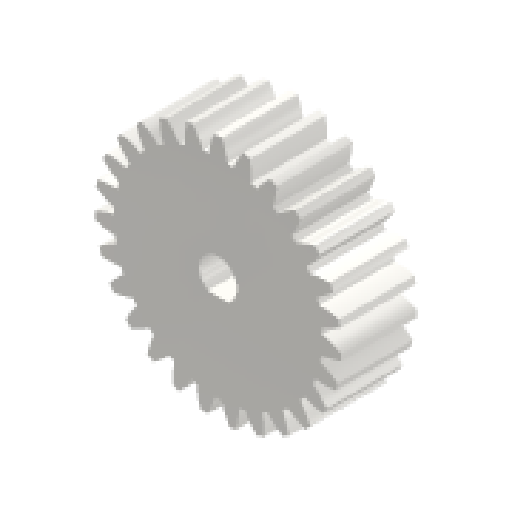
# Autodesk Inventor part: Stirnzahnrad1
Saved by Autodesk Inventor 2024.1 (Build 281209000, 209)
## iProperties
Created: 2024-04-15
Part Number: Stirnzahnrad1
Material: Steel
Document SubType Name: Modeling
Designer: diederichbenedict
Categories: <?xml version="1.0" encoding="UTF-16"?> <MemberInstance><Categories><FamilyTemplate><FamilyTemplateParameter ValueType="xs:double" Id="1" ObjectReferenceKey="da_z" ObjectType="kUserParameterObject"/><FamilyTemplateParameter ValueType="xs:double" Id="2" ObjectReferenceKey="da_b" ObjectType="kUserParameterObject"/><FamilyTemplateParameter ValueType="xs:double" Id="3" ObjectReferenceKey="da_beta" ObjectType="kUserParameterObject"/><FamilyTemplateParameter ValueType="xs:double" Id="4" ObjectReferenceKey="da_da" ObjectType="kUserParameterObject"/><FamilyTemplateParameter ValueType="xs:double" Id="5" ObjectReferenceKey="da_aw" ObjectType="kUserParameterObject"/><FamilyTemplateParameter ValueType="xs:string" Id="6" ObjectReferenceKey="EAIAABAAAACIAQAAAAAAAIAAAAAAAAAA" ObjectType="83910656" SubObjectId="SurfaceGeometry"/></FamilyTemplate><ParamToTemplateMap><ParamToTemplate CategoryParameter="//CategoryParameter[@InternalName='046C89C9-8512-4d59-83FE-43B91F4F132A']" TemplateParameter="1"/><ParamToTemplate CategoryParameter="//CategoryParameter[@InternalName='2552DF32-E462-4b46-AEBF-C6C7768E72AC']" TemplateParameter="2"/><ParamToTemplate CategoryParameter="//CategoryParameter[@InternalName='C9EE641D-15FC-4fae-A226-E94C4372FDD7']" TemplateParameter="3"/><ParamToTemplate><ParamToTemplate CategoryParameter="//CategoryParameter[@InternalName='00B6519A-459B-49c7-AD84-2E56D39A5744']" ConstantValue="0.000000"/></ParamToTemplate><ParamToTemplate><ParamToTemplate CategoryParameter="//CategoryParameter[@InternalName='04B31F0E-C7A6-4894-AA32-9629BEFACF47']" ConstantValue="1.000000"/></ParamToTemplate><ParamToTemplate><ParamToTemplate CategoryParameter="//CategoryParameter[@InternalName='43CBEC2E-7847-49e7-A936-2F7889FCB2D9']" ConstantValue="0.250000"/></ParamToTemplate><ParamToTemplate><ParamToTemplate CategoryParameter="//CategoryParameter[@InternalName='B1EFC894-105D-4ebd-86BF-FA20ED196853']" ConstantValue="0.350000"/></ParamToTemplate><ParamToTemplate><ParamToTemplate CategoryParameter="//CategoryParameter[@InternalName='51175063-3D10-4879-93E8-6246FE8B403D']" ConstantValue="2060000000.000000"/></ParamToTemplate><ParamToTemplate><ParamToTemplate CategoryParameter="//CategoryParameter[@InternalName='A3A52E27-4454-46a9-B0BD-C932399B70AF']" ConstantValue="0.300000"/></ParamToTemplate><ParamToTemplate><ParamToTemplate CategoryParameter="//CategoryParameter[@InternalName='91B76062-C214-41d9-B1B9-14D2AB99603D']" ConstantValue="0.112500"/></ParamToTemplate><ParamToTemplate><ParamToTemplate CategoryParameter="//CategoryParameter[@InternalName='374E806E-8B8A-4dda-A9AA-1039D6500AD2']" ConstantValue="8.888889"/></ParamToTemplate><ParamToTemplate><ParamToTemplate CategoryParameter="//CategoryParameter[@InternalName='2D373A89-B862-43d6-8D0B-0CBF12AB9F6C']" ConstantValue="0.349066"/></ParamToTemplate><ParamToTemplate CategoryParameter="//CategoryParameter[@InternalName='37777632-D6A2-4fac-9D53-DB8ACD95C989']" TemplateParameter="4"/><ParamToTemplate CategoryParameter="//CategoryParameter[@InternalName='FD1017F1-B727-4f7e-9707-0F86F1FF9423']" TemplateParameter="5"/><ParamToTemplate><ParamToTemplate CategoryParameter="//CategoryParameter[@InternalName='9E1B4470-B2D3-4ff1-B813-535BB4CDF51A']" ConstantValue="3520000.000000"/></ParamToTemplate><ParamToTemplate><ParamToTemplate CategoryParameter="//CategoryParameter[@InternalName='F8452263-BFF6-458c-9FB1-07C4B99E95CD']" ConstantValue="11400000.000000"/></ParamToTemplate><ParamToTemplate><ParamToTemplate CategoryParameter="//CategoryParameter[@InternalName='3E3BB259-FD49-497f-8171-6EBC954A3479']" ConstantValue="2.000000"/></ParamToTemplate><ParamToTemplate CategoryParameter="//CategoryParameter[@InternalName='27C3BAF2-7550-4e4b-AE2C-0DB134B7D9B7']" TemplateParameter="6"/></ParamToTemplateMap><Category DisplayName="Gear" InternalName="DC85795E-93AB-48d5-8EEE-5A27447B64BD" Mnemonic="Gear"><CategoryParameter DisplayName="z" InternalName="046C89C9-8512-4d59-83FE-43B91F4F132A" Mnemonic="z"/><CategoryParameter DisplayName="b" InternalName="2552DF32-E462-4b46-AEBF-C6C7768E72AC" Mnemonic="b"/><CategoryParameter DisplayName="||b|" InternalName="C9EE641D-15FC-4fae-A226-E94C4372FDD7" Mnemonic="beta"/><CategoryParameter DisplayName="x" InternalName="00B6519A-459B-49c7-AD84-2E56D39A5744" Mnemonic="x"/><CategoryParameter DisplayName="a*" InternalName="04B31F0E-C7A6-4894-AA32-9629BEFACF47" Mnemonic="a"/><CategoryParameter DisplayName="c*" InternalName="43CBEC2E-7847-49e7-A936-2F7889FCB2D9" Mnemonic="c"/><CategoryParameter DisplayName="r|.f|*" InternalName="B1EFC894-105D-4ebd-86BF-FA20ED196853" Mnemonic="rf"/><CategoryParameter DisplayName="E" InternalName="51175063-3D10-4879-93E8-6246FE8B403D" Mnemonic="E"/><CategoryParameter DisplayName="||m|" InternalName="A3A52E27-4454-46a9-B0BD-C932399B70AF" Mnemonic="mi"/><Category DisplayName="SpurGear" InternalName="26C5A22E-A91E-4dfd-A3B3-23CCAFAE1764" Mnemonic="SpurGear"><CategoryParameter DisplayName="m" InternalName="91B76062-C214-41d9-B1B9-14D2AB99603D" Mnemonic="m"/><CategoryParameter DisplayName="P" InternalName="374E806E-8B8A-4dda-A9AA-1039D6500AD2" Mnemonic="PP"/><CategoryParameter DisplayName="||a|" InternalName="2D373A89-B862-43d6-8D0B-0CBF12AB9F6C" Mnemonic="alpha"/><CategoryParameter DisplayName="d|.a|" InternalName="37777632-D6A2-4fac-9D53-DB8ACD95C989" Mnemonic="da"/><CategoryParameter DisplayName="a|.w|" InternalName="FD1017F1-B727-4f7e-9707-0F86F1FF9423" Mnemonic="aw"/><CategoryParameter DisplayName="||s||.Flim|" InternalName="9E1B4470-B2D3-4ff1-B813-535BB4CDF51A" Mnemonic="sFlim"/><CategoryParameter DisplayName="||s||.Hlim|" InternalName="F8452263-BFF6-458c-9FB1-07C4B99E95CD" Mnemonic="sHlim"/><CategoryParameter DisplayName="Typ" InternalName="3E3BB259-FD49-497f-8171-6EBC954A3479" Mnemonic="type"/><CategoryParameter DisplayName="PitchDiameter" InternalName="27C3BAF2-7550-4e4b-AE2C-0DB134B7D9B7" Mnemonic="IDS_PITCHDIAM"/></Category></Category></Categories></MemberInstance>
Density: 1 g/cm^3
Appearance: Steel
CustomPartVersion: 1
Author: diederichbenedict
Autodesk Inventor part; units mm, degrees
sketch "Sketch1" plane through (0, 0, 0) normal (0, 0, 1) x (1, 0, 0)
  circle A0 centre (0, 0) radius 16.3108
  dimension "d0" = 32.6217
  constraints: 1 centre point
  measures "d0" diameter of A0
extrude "Extrusion1" add sketch "Sketch1" along normal blind 10
ref_plane "Work Plane2" through (0, 0, 5) normal (0, 0, 1) x (1, 0, 0)
sketch "Sketch2" plane through (0, 0, 0) normal (0, 0, -1) x (-1, 0, 0)
  circle A0 centre (0, 0) radius 16.3108 projected
  circle A1 centre (0, 0) radius 15.1875
  dimension "d3" = 30.375
  constraints: 1 centre point, 1 coincident
  measures "d3" diameter of A1
surface extrude "Flankendurchmesser" sketch "Sketch2" against normal through all shown no curves A1
ref_plane "Work Plane8" through (0, 0, 0) normal (0.9932384, 0.1160929, 0) x (0, 0, 1)
ref_plane "Work Plane9" through (0, 0, 0) normal (1, 0, 0) x (0, 1, 0)
spur gear teeth "Stirnzahnrad" teeth 27 pitch diameter 30.375 tip diameter 32.6217 root diameter 27.5625 face width 20 start plane through (0, 0, 0) normal (0, 0, -1) x (-1, 0, 0)
sketch "Skizze3" plane through (0, 0, 10) normal (0, 0, 1) x (1, 0, 0)
  arc A0 (-4.2216, 15.7551) -> (-4.3348, 13.0818) centre (6.3804, 13.9668) ccw projected
  arc A1 (-4.3348, 13.0818) -> (-5.0881, 12.8076) centre (0, 0) ccw projected
  arc A2 (-5.0881, 12.8076) -> (-6.8933, 14.7826) centre (-13.8653, 6.598) ccw projected
  arc A3 (-6.8933, 14.7826) -> (-7.7411, 14.3568) centre (0, 0) ccw projected
  arc A4 (-7.7411, 14.3568) -> (-7.2348, 11.7295) centre (2.9874, 15.0617) ccw projected
  arc A5 (-7.2348, 11.7295) -> (-7.9046, 11.2889) centre (0, 0) ccw projected
  arc A6 (-7.9046, 11.2889) -> (-10.1166, 12.7945) centre (-15.0132, 3.2225) ccw projected
  arc A7 (-10.1166, 12.7945) -> (-10.8434, 12.1846) centre (0, 0) ccw projected
  arc A8 (-10.8434, 12.1846) -> (-9.7448, 9.7448) centre (-0.5666, 15.3447) ccw projected
  arc A9 (-9.7448, 9.7448) -> (-10.2949, 9.1617) centre (0, 0) ccw projected
  arc A10 (-10.2949, 9.1617) -> (-12.7945, 10.1166) centre (-15.3517, -0.3266) ccw projected
  arc A11 (-12.7945, 10.1166) -> (-13.361, 9.3555) centre (0, 0) ccw projected
  arc A12 (-13.361, 9.3555) -> (-11.7295, 7.2348) centre (-4.09, 14.8004) ccw projected
  arc A13 (-11.7295, 7.2348) -> (-12.1303, 6.5406) centre (0, 0) ccw projected
  arc A14 (-12.1303, 6.5406) -> (-14.7826, 6.8933) centre (-14.8626, -3.8581) ccw projected
  arc A15 (-14.7826, 6.8933) -> (-15.1584, 6.0221) centre (0, 0) ccw projected
  arc A16 (-15.1584, 6.0221) -> (-13.0818, 4.3348) centre (-7.393, 13.4583) ccw projected
  arc A17 (-13.0818, 4.3348) -> (-13.3117, 3.5668) centre (0, 0) ccw projected
  arc A18 (-13.3117, 3.5668) -> (-15.9739, 3.2983) centre (-13.5722, -7.1817) ccw projected
  arc A19 (-15.9739, 3.2983) -> (-16.1386, 2.364) centre (0, 0) ccw projected
  arc A20 (-16.1386, 2.364) -> (-13.7288, 1.2011) centre (-10.2974, 11.3905) ccw projected
  arc A21 (-13.7288, 1.2011) -> (-13.7754, 0.4008) centre (0, 0) ccw projected
  arc A22 (-13.7754, 0.4008) -> (-16.3039, -0.4744) centre (-11.5501, -10.1181) ccw projected
  arc A23 (-16.3039, -0.4744) -> (-16.2488, -1.4216) centre (0, 0) ccw projected
  arc A24 (-16.2488, -1.4216) -> (-13.6357, -1.9973) centre (-12.6467, 8.7088) ccw projected
  arc A25 (-13.6357, -1.9973) -> (-13.4965, -2.7868) centre (0, 0) ccw projected
  arc A26 (-13.4965, -2.7868) -> (-15.7551, -4.2216) centre (-8.9054, -12.509) ccw projected
  arc A27 (-15.7551, -4.2216) -> (-15.4829, -5.1305) centre (0, 0) ccw projected
  arc A28 (-15.4829, -5.1305) -> (-12.8076, -5.0881) centre (-14.3142, 5.5575) ccw projected
  arc A29 (-12.8076, -5.0881) -> (-12.4901, -5.8242) centre (0, 0) ccw projected
  arc A30 (-12.4901, -5.8242) -> (-14.3568, -7.7411) centre (-5.7806, -14.2255) ccw projected
  arc A31 (-14.3568, -7.7411) -> (-13.8824, -8.5628) centre (0, 0) ccw projected
  arc A32 (-13.8824, -8.5628) -> (-11.2889, -7.9046) centre (-15.21, 2.1066) ccw projected
  arc A33 (-11.2889, -7.9046) -> (-10.8102, -8.5476) centre (0, 0) ccw projected
  arc A34 (-10.8102, -8.5476) -> (-12.1846, -10.8434) centre (-2.3441, -15.1752) ccw projected
  arc A35 (-12.1846, -10.8434) -> (-11.5335, -11.5335) centre (0, 0) ccw projected
  arc A36 (-11.5335, -11.5335) -> (-9.1617, -10.2949) centre (-15.2858, -1.4578) ccw projected
  arc A37 (-9.1617, -10.2949) -> (-8.5476, -10.8102) centre (0, 0) ccw projected
  arc A38 (-8.5476, -10.8102) -> (-9.3555, -13.361) centre (1.2187, -15.3067) ccw projected
  arc A39 (-9.3555, -13.361) -> (-8.5628, -13.8824) centre (0, 0) ccw projected
  arc A40 (-8.5628, -13.8824) -> (-6.5406, -12.1303) centre (-14.5376, -4.9437) ccw projected
  arc A41 (-6.5406, -12.1303) -> (-5.8242, -12.4901) centre (0, 0) ccw projected
  arc A42 (-5.8242, -12.4901) -> (-6.0221, -15.1584) centre (4.7158, -14.6131) ccw projected
  arc A43 (-6.0221, -15.1584) -> (-5.1305, -15.4829) centre (0, 0) ccw projected
  arc A44 (-5.1305, -15.4829) -> (-3.5668, -13.3117) centre (-13.0056, -8.163) ccw projected
  arc A45 (-3.5668, -13.3117) -> (-2.7868, -13.4965) centre (0, 0) ccw projected
  arc A46 (-2.7868, -13.4965) -> (-2.364, -16.1386) centre (7.9587, -13.1316) ccw projected
  arc A47 (-2.364, -16.1386) -> (-1.4216, -16.2488) centre (0, 0) ccw projected
  arc A48 (-1.4216, -16.2488) -> (-0.4008, -13.7754) centre (-10.7725, -10.9423) ccw projected
  arc A49 (-0.4008, -13.7754) -> (0.4008, -13.7754) centre (0, 0) ccw projected
  arc A50 (0.4008, -13.7754) -> (1.4216, -16.2488) centre (10.7725, -10.9423) ccw projected
  arc A51 (1.4216, -16.2488) -> (2.364, -16.1386) centre (0, 0) ccw projected
  arc A52 (2.364, -16.1386) -> (2.7868, -13.4965) centre (-7.9587, -13.1316) ccw projected
  arc A53 (2.7868, -13.4965) -> (3.5668, -13.3117) centre (0, 0) ccw projected
  arc A54 (3.5668, -13.3117) -> (5.1305, -15.4829) centre (13.0056, -8.163) ccw projected
  arc A55 (5.1305, -15.4829) -> (6.0221, -15.1584) centre (0, 0) ccw projected
  arc A56 (6.0221, -15.1584) -> (5.8242, -12.4901) centre (-4.7158, -14.6131) ccw projected
  arc A57 (5.8242, -12.4901) -> (6.5406, -12.1303) centre (0, 0) ccw projected
  arc A58 (6.5406, -12.1303) -> (8.5628, -13.8824) centre (14.5376, -4.9437) ccw projected
  arc A59 (8.5628, -13.8824) -> (9.3555, -13.361) centre (0, 0) ccw projected
  arc A60 (9.3555, -13.361) -> (8.5476, -10.8102) centre (-1.2187, -15.3067) ccw projected
  arc A61 (8.5476, -10.8102) -> (9.1617, -10.2949) centre (0, 0) ccw projected
  arc A62 (9.1617, -10.2949) -> (11.5335, -11.5335) centre (15.2858, -1.4578) ccw projected
  arc A63 (11.5335, -11.5335) -> (12.1846, -10.8434) centre (0, 0) ccw projected
  arc A64 (12.1846, -10.8434) -> (10.8102, -8.5476) centre (2.3441, -15.1752) ccw projected
  arc A65 (10.8102, -8.5476) -> (11.2889, -7.9046) centre (0, 0) ccw projected
  arc A66 (11.2889, -7.9046) -> (13.8824, -8.5628) centre (15.21, 2.1066) ccw projected
  arc A67 (13.8824, -8.5628) -> (14.3568, -7.7411) centre (0, 0) ccw projected
  arc A68 (14.3568, -7.7411) -> (12.4901, -5.8242) centre (5.7806, -14.2255) ccw projected
  arc A69 (12.4901, -5.8242) -> (12.8076, -5.0881) centre (0, 0) ccw projected
  arc A70 (12.8076, -5.0881) -> (15.4829, -5.1305) centre (14.3142, 5.5575) ccw projected
  arc A71 (15.4829, -5.1305) -> (15.7551, -4.2216) centre (0, 0) ccw projected
  arc A72 (15.7551, -4.2216) -> (13.4965, -2.7868) centre (8.9054, -12.509) ccw projected
  arc A73 (13.4965, -2.7868) -> (13.6357, -1.9973) centre (0, 0) ccw projected
  arc A74 (13.6357, -1.9973) -> (16.2488, -1.4216) centre (12.6467, 8.7088) ccw projected
  arc A75 (16.2488, -1.4216) -> (16.3039, -0.4744) centre (0, 0) ccw projected
  arc A76 (16.3039, -0.4744) -> (13.7754, 0.4008) centre (11.5501, -10.1181) ccw projected
  arc A77 (13.7754, 0.4008) -> (13.7288, 1.2011) centre (0, 0) ccw projected
  arc A78 (13.7288, 1.2011) -> (16.1386, 2.364) centre (10.2974, 11.3905) ccw projected
  arc A79 (16.1386, 2.364) -> (15.9739, 3.2983) centre (0, 0) ccw projected
  arc A80 (15.9739, 3.2983) -> (13.3117, 3.5668) centre (13.5722, -7.1817) ccw projected
  arc A81 (13.3117, 3.5668) -> (13.0818, 4.3348) centre (0, 0) ccw projected
  arc A82 (13.0818, 4.3348) -> (15.1584, 6.0221) centre (7.393, 13.4583) ccw projected
  arc A83 (15.1584, 6.0221) -> (14.7826, 6.8933) centre (0, 0) ccw projected
  arc A84 (14.7826, 6.8933) -> (12.1303, 6.5406) centre (14.8626, -3.8581) ccw projected
  arc A85 (12.1303, 6.5406) -> (11.7295, 7.2348) centre (0, 0) ccw projected
  arc A86 (11.7295, 7.2348) -> (13.361, 9.3555) centre (4.09, 14.8004) ccw projected
  arc A87 (13.361, 9.3555) -> (12.7945, 10.1166) centre (0, 0) ccw projected
  arc A88 (12.7945, 10.1166) -> (10.2949, 9.1617) centre (15.3517, -0.3266) ccw projected
  arc A89 (10.2949, 9.1617) -> (9.7448, 9.7448) centre (0, 0) ccw projected
  arc A90 (9.7448, 9.7448) -> (10.8434, 12.1846) centre (0.5666, 15.3447) ccw projected
  arc A91 (10.8434, 12.1846) -> (10.1166, 12.7945) centre (0, 0) ccw projected
  arc A92 (10.1166, 12.7945) -> (7.9046, 11.2889) centre (15.0132, 3.2225) ccw projected
  arc A93 (7.9046, 11.2889) -> (7.2348, 11.7295) centre (0, 0) ccw projected
  arc A94 (7.2348, 11.7295) -> (7.7411, 14.3568) centre (-2.9874, 15.0617) ccw projected
  arc A95 (7.7411, 14.3568) -> (6.8933, 14.7826) centre (0, 0) ccw projected
  arc A96 (6.8933, 14.7826) -> (5.0881, 12.8076) centre (13.8653, 6.598) ccw projected
  arc A97 (5.0881, 12.8076) -> (4.3348, 13.0818) centre (0, 0) ccw projected
  arc A98 (4.3348, 13.0818) -> (4.2216, 15.7551) centre (-6.3804, 13.9668) ccw projected
  arc A99 (4.2216, 15.7551) -> (3.2983, 15.9739) centre (0, 0) ccw projected
  arc A100 (3.2983, 15.9739) -> (1.9973, 13.6357) centre (11.97, 9.6177) ccw projected
  arc A101 (1.9973, 13.6357) -> (1.2011, 13.7288) centre (0, 0) ccw projected
  arc A102 (1.2011, 13.7288) -> (0.4744, 16.3039) centre (-9.4294, 12.1189) ccw projected
  arc A103 (0.4744, 16.3039) -> (-0.4744, 16.3039) centre (0, 0) ccw projected
  arc A104 (-0.4744, 16.3039) -> (-1.2011, 13.7288) centre (9.4294, 12.1189) ccw projected
  arc A105 (-1.2011, 13.7288) -> (-1.9973, 13.6357) centre (0, 0) ccw projected
  arc A106 (-1.9973, 13.6357) -> (-3.2983, 15.9739) centre (-11.97, 9.6177) ccw projected
  arc A107 (-3.2983, 15.9739) -> (-4.2216, 15.7551) centre (0, 0) ccw projected
  circle A108 centre (0, 0) radius 2.5
  line L0 (-1.3565, -2.1) -> (1.3565, -2.1)
  point P0 (0, -2.1)
  dimension "d49" = 5
  dimension "d52" = 2.1
  constraints: 2 end point, 2 point on circle, 1 centre point, 1 coincident, 1 horizontal, 1 midpoint
  measures "d49" diameter of A108
  measures "d52" distance of point (0, -2.1) point (0, 0)
extrude "Extrusion2" cut sketch "Skizze3" against normal through all contours A108 L0 picked at (0.6245, 0.1306)
chamfer "Fasen1" distance 1 angle 45 4 edges at (0, 2.5, 0) (0, 2.5, 10) (0, -2.1, 10) (0, -2.1, 0)
equation "\"d0\" = da_da"
equation "\"d3\" = da_d"
equation "\"d16\" = da_aw"
equation "\"d43\" = da_aw"
equation "\"d46\" = da_aw"
equation "\"da_da\" = 32.62166"
equation "\"da_d\" = 30.375"
equation "\"da_aw\" = 35"
body "Solid1"
body "Srf1"
